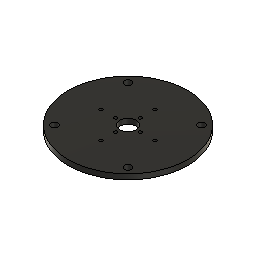
Winch1 (Autodesk Fusion 360 design; units mm, degrees)
Autodesk Fusion 360 part; units mm, degrees
sketch "Sketch1" plane through (0, 0, 0) normal (0, 0, 1) x (1, 0, 0)
  circle A0 centre (0, 0) radius 7.5
  circle A1 centre (16.5, 0) radius 0.9375
  circle A2 centre (-16.5, 0) radius 0.9375
  circle A3 centre (0, -16.5) radius 0.9375
  circle A4 centre (0, 16.5) radius 0.9375
  line L0 (0, 0) -> (18.2563, 0) construction
  circle A5 centre (22.4506, 22.4506) radius 2.159
  circle A6 centre (22.4506, -22.4506) radius 2.159
  circle A7 centre (-22.4506, -22.4506) radius 2.159
  circle A8 centre (-22.4506, 22.4506) radius 2.159
  circle A9 centre (0, 0) radius 5
  circle A10 centre (0, 0) radius 36.5125
  line L1 (0, 0) -> (22.4506, 22.4506)
  line L2 (0, 0) -> (21.082, 0) construction
  line L3 (0, 0) -> (22.4506, -22.4506)
  line L4 (0, 0) -> (21.082, 0) construction
  line L5 (0, 0) -> (-22.4506, -22.4506)
  line L6 (0, 0) -> (21.082, 0) construction
  line L7 (0, 0) -> (-22.4506, 22.4506)
  line L8 (0, 0) -> (21.082, 0) construction
  arc A11 (-20.873, 23.9245) -> (20.873, 23.9245) centre (0, 0) ccw
  line L9 (16.5, 0) -> (10.5, 0)
  circle A12 centre (0, 0) radius 5.2451
  circle A13 centre (7.5, 0) radius 0.9375
  circle A14 centre (0, 7.5) radius 0.9375
  circle A15 centre (-7.5, 0) radius 0.9375
  circle A16 centre (0, -7.5) radius 0.9375
  dimension "d2" = 15
  dimension "d6" = 1.875
  dimension "d7" = 1.875
  dimension "d8" = 1.875
  dimension "d9" = 1.875
  dimension "d16" = 4.318
  dimension "d17" = 4.318
  dimension "d18" = 4.318
  dimension "d19" = 4.318
  dimension "d21" = 10
  dimension "d24" = 73.025
  dimension "d25" = 63.5
  dimension "d26" = 45
  dimension "d27" = 45
  dimension "d28" = 135
  dimension "d29" = 135
  dimension "d31" = 6
  dimension "d32" = 10.4902
  dimension "d33" = 1.875
  dimension "d35" = 360
  constraint coincident A0.centre L0.start
  constraint horizontal L0
  constraint concentric A10 A11
  constraint horizontal L2
  constraint coincident A5.centre A11
  constraint coincident A5.centre L1.end
  constraint horizontal L4
  constraint coincident A6.centre A11
  constraint coincident A6.centre L3.end
  constraint horizontal L6
  constraint coincident A7.centre A11
  constraint coincident A7.centre L5.end
  constraint horizontal L8
  constraint coincident A8.centre A11
  constraint coincident A8.centre L7.end
  constraint coincident A5 A11.end
  constraint coincident A8 A11.start
  constraint coincident A1.centre L9.start
  constraint coincident L0 L9.end
  constraint coincident L6 L9.end
  constraint concentric A0 A12
  constraint coincident L2 A13.centre
  constraint coincident A0 A13.centre
  measures "d2" diameter of A0
  measures "d6" diameter of A1
  measures "d7" diameter of A2
  measures "d8" diameter of A3
  measures "d9" diameter of A4
  measures "d16" diameter of A5
  measures "d17" diameter of A6
  measures "d18" diameter of A7
  measures "d19" diameter of A8
  measures "d21" diameter of A9
  measures "d24" diameter of A10
  measures "d25" diameter of A11
  measures "d26" angle of L1 L2
  measures "d27" angle of L3 L4
  measures "d28" angle of L5 L6
  measures "d29" angle of L7 L8
  measures "d31" distance of A1.centre L9.end
  measures "d32" diameter of A12
  measures "d33" diameter of A13
extrude "Extrude1" add sketch "Sketch1" along normal blind 3.175 contours A0 L1 L3 A12 A13 | A0 A5 A6 L1 L3 A11 A13 | A0 L1 L7 A12 A14 | A0 A6 A7 L3 L5 A11 A16 | A0 L3 L5 A12 A16 | A9 L1 L3 A12 | A9 L1 L7 A12 | A9 L3 L5 A12 | A0 L5 L7 A12 A15 | A9 L5 L7 A12 | A0 A7 A8 L5 L7 A11 A15 | A10
equation "d22 = ( 1 / 8 ) * 1 in"
named bodies: "Winch1"
